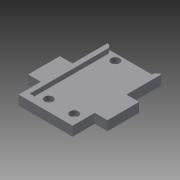
# Autodesk Inventor part: soporte
Saved by Autodesk Inventor 2015 SP1 (Build 190203100, 203)
## iProperties
Created: 2015-06-09
Part Number: soporte
Material: Generic
Document SubType Name: Modeling
Designer: pc
Density: 1 g/cm^3
Appearance: Default
Author: pc
Autodesk Inventor part; units mm, degrees
ref_plane "YZ Plane" through (0, 0, 0) normal (1, 0, 0) x (0, 1, 0)
ref_plane "XZ Plane" through (0, 0, 0) normal (0, 1, 0) x (-1, 0, 0)
ref_plane "XY Plane" through (0, 0, 0) normal (0, 0, 1) x (1, 0, 0)
sketch "Sketch1" plane through (0, 0, 0) normal (0, 0, 1) x (1, 0, 0)
  line L0 (-17, 28) -> (0, 28)
  line L1 (4, 7) -> (0, 7)
  line L2 (0, 7) -> (0, 0)
  line L3 (0, 0) -> (-17, 0)
  line L4 (-17, 0) -> (-17, 7)
  line L5 (-17, 28) -> (-17, 17)
  line L6 (-17, 17) -> (-21, 17)
  line L7 (-21, 17) -> (-21, 7)
  line L8 (-21, 7) -> (-17, 7)
  line L9 (0, 28) -> (0, 17)
  line L10 (0, 17) -> (4, 17)
  line L11 (4, 17) -> (4, 7)
  point P0 (0, 0)
  dimension "d0" = 17
  dimension "d1" = 10
  dimension "d2" = 28
  dimension "d3" = 4
  dimension "d6" = 7
  constraints: 24 end point, 6 perpendicular, 4 collinear, 4 point on line, 2 coincident, 2 vertical, 2 other
  measures "d0" distance of L0.start L0.end
  measures "d1" distance of L6.end L7.end
  measures "d2" distance between parallel lines of L3 L0
  measures "d3" distance of L5.end L6.end
  measures "d6" distance of L3.end L4.end
extrude "Extrusion1" add sketch "Sketch1" along normal blind 3
sketch "Sketch2" plane through (0, 0, 3) normal (0, 0, 1) x (1, 0, 0)
  line L0 (-17, 28) -> (-17, 17) projected
  line L1 (-17, 17) -> (-21, 17) projected
  line L2 (-21, 17) -> (-21, 7) projected
  line L3 (-21, 7) -> (-17, 7) projected
  line L4 (-17, 7) -> (-17, 0) projected
  line L5 (-17, 0) -> (0, 0) projected
  line L6 (0, 0) -> (0, 7) projected
  line L7 (0, 7) -> (4, 7) projected
  line L8 (4, 7) -> (4, 17) projected
  line L9 (4, 17) -> (0, 17) projected
  line L10 (0, 17) -> (0, 28) projected
  line L11 (0, 28) -> (-17, 28) projected
  line L12 (-17, 0) -> (0, 0) projected
  line L13 (-15.5, 2) -> (-1.5, 2)
  line L14 (-1.5, 2) -> (-1.5, 28)
  line L15 (-1.5, 28) -> (-15.5, 28)
  line L16 (-15.5, 28) -> (-15.5, 2)
  line L17 (0, 28) -> (-17, 28) projected
  dimension "d7" = 14
  dimension "d8" = 1.5
  dimension "d19" = 26
  constraints: 8 end point, 2 parallel, 1 horizontal, 1 perpendicular, 1 point on line
  measures "d7" distance of L15.end L14.end
  measures "d8" distance between parallel lines of L4 L16
  measures "d19" distance of L13.end L14.end
extrude "Extrusion2" cut sketch "Sketch2" against normal blind 1.5 contours L11 L14 L13 L16
sketch "Sketch3" plane through (0, 0, 1.5) normal (0, 0, 1) x (1, 0, 0)
  line L0 (-1.5, 28) -> (-1.5, 2) projected
  line L1 (-15.5, 28) -> (-1.5, 28) projected
  line L2 (-15.5, 2) -> (-15.5, 28) projected
  circle A0 centre (-12.5, 26) radius 1.35
  circle A1 centre (-12.5, 5) radius 1.35
  circle A2 centre (-4.5, 5) radius 1.35
  line L3 (-1.5, 2) -> (-15.5, 2) projected
  point P0 (0, 0)
  dimension "d12" = 2.7
  dimension "d13" = 8
  dimension "d14" = 21
  dimension "d21" = 3
  constraints: 3 centre point, 2 equal radius, 1 horizontal alignment, 1 vertical alignment
  measures "d12" diameter of A1
  measures "d13" distance of A2.centre A1.centre
  measures "d14" distance of A1.centre A0.centre
  measures "d21" distance from line of L3 A1.centre
extrude "Extrusion3" cut sketch "Sketch3" against normal through all contours A0 | A1 | A2
fillet "Fillet1" radius 1.5 2 edges at (-15.5, 28, 2.25) (-1.5, 28, 2.25)
body "Solid1"
